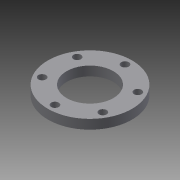
# Autodesk Inventor part: Rough_Spacer
Saved by Autodesk Inventor 2014 SP1 (Build 180222100, 222)
## iProperties
Created: 2014-04-03
Part Number: Rough_Spacer
Material: Generic
Document SubType Name: Modeling
Designer: carpenma
Density: 1 g/cm^3
Appearance: Default
Author: carpenma
Autodesk Inventor part; units mm, degrees
ref_plane "YZ Plane" through (0, 0, 0) normal (1, 0, 0) x (0, 1, 0)
ref_plane "XZ Plane" through (0, 0, 0) normal (0, 1, 0) x (-1, 0, 0)
ref_plane "XY Plane" through (0, 0, 0) normal (0, 0, 1) x (1, 0, 0)
sketch "Sketch1" plane through (0, 0, 0) normal (0, 1, 0) x (-1, 0, 0)
  circle A0 centre (0, 0) radius 28.575
  circle A1 centre (0, 0) radius 15.875
  dimension "d0" = 57.15
  dimension "d1" = 31.75
  constraints: 2 centre point, 2 coincident
  measures "d0" diameter of A0
  measures "d1" diameter of A1
extrude "Extrusion1" add sketch "Sketch1" against normal blind 6.35
sketch "Sketch2" plane through (0, 0, 0) normal (0, 1, 0) x (1, 0, 0)
  circle A0 centre (0, 0) radius 28.575 projected
  circle A1 centre (0, 0) radius 23.8125
  circle A2 centre (0, 23.8125) radius 2.5908
  circle A3 centre (-20.6222, 11.9063) radius 2.5908
  circle A4 centre (-20.6222, -11.9062) radius 2.5908
  circle A5 centre (0, -23.8125) radius 2.5908
  circle A6 centre (20.6222, -11.9063) radius 2.5908
  circle A7 centre (20.6222, 11.9062) radius 2.5908
  dimension "d4" = 47.625
  dimension "d5" = 5.1816
  dimension "d8" = 360
  constraints: 6 centre point, 1 coincident, 1 vertical alignment, 15 other
  measures "d5" diameter of A2
extrude "Extrusion2" cut sketch "Sketch2" against normal blind 25.4 contours A7 A1 | A1 A7 | A6 A1 | A1 A6 | A2 A1 | A1 A2 | A5 A1 | A1 A5 | A3 A1 | A1 A3 | A4 A1 | A1 A4
body "Solid1"
